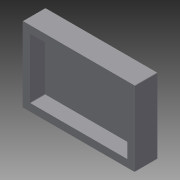
# Autodesk Inventor part: Panel_Body
Saved by Autodesk Inventor 2013 (Build 170138000, 138)
## iProperties
Created: 2013-01-11
Part Number: Panel_Body
Material: Generic
Document SubType Name: Modeling
Designer: mstine
Density: 1 g/cm^3
Author: mstine
Autodesk Inventor part; units mm, degrees
ref_plane "YZ Plane" through (0, 0, 0) normal (1, 0, 0) x (0, 1, 0)
ref_plane "XZ Plane" through (0, 0, 0) normal (0, 1, 0) x (-1, 0, 0)
ref_plane "XY Plane" through (0, 0, 0) normal (0, 0, 1) x (1, 0, 0)
sketch "PanelDimension" plane through (0, 0, 0) normal (0, 0, 1) x (1, 0, 0)
  line L0 (-187.5, 125) -> (187.5, 125)
  line L1 (187.5, 125) -> (187.5, -125)
  line L2 (187.5, -125) -> (-187.5, -125)
  line L3 (-187.5, -125) -> (-187.5, 125)
  point P0 (0, 0)
  point P1 (-187.5, 0)
  point P2 (0, 125)
  dimension "d0" = 375
  dimension "d2" = 250
  constraints: 8 end point, 2 midpoint, 2 parallel, 1 horizontal, 1 horizontal alignment, 1 perpendicular, 1 vertical alignment
  measures "d0" distance of L0.start L0.end
  measures "d2" distance of L2.end L0.start
extrude "BodyExtrusion" add sketch "PanelDimension" along normal blind 75
sketch "PanelInside" plane through (0, 0, 75) normal (0, 0, 1) x (1, 0, 0)
  line L0 (187.5, 125) -> (-187.5, 125) projected
  line L1 (-187.5, 125) -> (-187.5, -125) projected
  line L2 (-162.5, 100) -> (162.5, 100)
  line L3 (162.5, 100) -> (162.5, -100)
  line L4 (162.5, -100) -> (-162.5, -100)
  line L5 (-162.5, -100) -> (-162.5, 100)
  point P0 (0, 0)
  point P1 (-162.5, 0)
  point P2 (0, 100)
  dimension "d7" = 25
  dimension "d8" = 25
  constraints: 8 end point, 2 midpoint, 2 parallel, 1 horizontal, 1 horizontal alignment, 1 perpendicular, 1 vertical alignment
  measures "d7" distance between parallel lines of L5 L1
  measures "d8" distance between parallel lines of L0 L2
extrude "CavityExtrusion" cut sketch "PanelInside" against normal blind 50
fillet "BodyOutsideFillet" radius 2 4 edges at (-187.5, 125, 37.5) (187.5, 125, 37.5) (187.5, -125, 37.5) (-187.5, -125, 37.5)
fillet "BodyInsideFillet" radius 2 4 edges at (162.5, 100, 50) (-162.5, 100, 50) (-162.5, -100, 50) (162.5, -100, 50)
body "Solid1"
